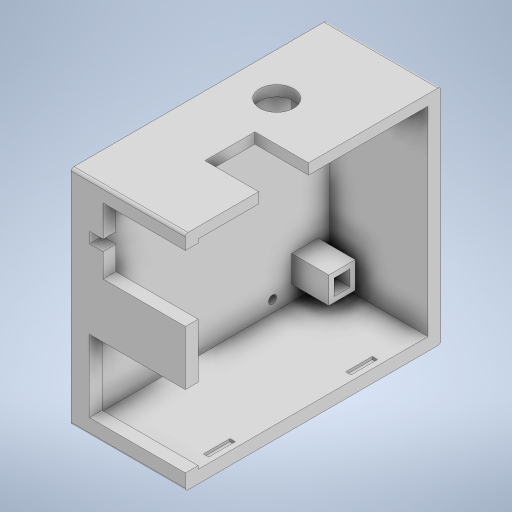
# Autodesk Inventor part: Enclosure_Top_v2
Saved by Autodesk Inventor 2023 (Build 270158030, 158C)
## iProperties
Created: 2023-12-07
Part Number: Enclosure_Top_v2
Material: Generic
Document SubType Name: Sheet Metal
Designer: Fabian
Density: 1 g/cm^3
Sheet Metal Rule: Default_mm
Appearance: Default
Author: Fabian
Autodesk Inventor part; units mm, degrees
ref_plane "YZ Plane" through (0, 0, 0) normal (1, 0, 0) x (0, 1, 0)
ref_plane "XZ Plane" through (0, 0, 0) normal (0, 1, 0) x (-1, 0, 0)
ref_plane "XY Plane" through (0, 0, 0) normal (0, 0, 1) x (1, 0, 0)
sketch "Sketch1" plane through (0, 0, 0) normal (1, 0, 0) x (0, 1, 0)
  line L0 (10.2141, 17.9541) -> (-31.7859, 17.9541)
  line L1 (-31.7859, 17.9541) -> (-31.7859, -30.1559)
  line L2 (-31.7859, -30.1559) -> (10.2141, -30.1559)
  line L3 (10.2141, -30.1559) -> (10.2141, 17.9541)
  point P0 (0, 0)
  dimension "d0" = 42
  dimension "d1" = 48.11
  constraints: 8 end point, 2 parallel, 1 horizontal, 1 perpendicular
  measures "d0" distance of L2.end L1.end
  measures "d1" distance of L1.end L0.end
extrude "BasePlate" add sketch "Sketch1" along normal blind 3
sketch "Sketch2" plane through (3, 0, 0) normal (1, 0, 0) x (0, 0, -1)
  point P0 (0, 0)
sketch "Sketch3" plane through (3, 0, 0) normal (1, 0, 0) x (0, 0, -1)
  line L0 (30.1559, 10.2141) -> (-17.9541, 10.2141) projected
  line L1 (-17.9541, -31.7859) -> (30.1559, -31.7859) projected
  line L2 (-17.9541, 10.2141) -> (30.1559, 10.2141)
  line L3 (30.1559, 10.2141) -> (30.1559, -31.7859)
  line L4 (30.1559, -31.7859) -> (-17.9541, -31.7859)
  line L5 (-17.9541, -31.7859) -> (-17.9541, 10.2141)
  line L6 (-15.5541, 8.2141) -> (27.7559, 8.2141)
  line L7 (27.7559, 8.2141) -> (27.7559, -29.3859)
  line L8 (27.7559, -29.3859) -> (-15.5541, -29.3859)
  line L9 (-15.5541, -29.3859) -> (-15.5541, 8.2141)
  point P0 (0, 0)
  point P1 (-17.9541, -10.7859)
  dimension "d4" = 2
  dimension "d5" = 2.4
  dimension "d6" = 2.4
  dimension "d7" = 2.4
  constraints: 16 end point, 4 parallel, 2 horizontal, 2 perpendicular, 1 midpoint
  measures "d4" distance between parallel lines of L0 L6
  measures "d5" distance between parallel lines of L1 L8
  measures "d6" distance from line of point (-17.954, -10.786) L9
  measures "d7" distance between parallel lines of L3 L7
extrude "Walls" add sketch "Sketch3" along normal blind 18.5
sketch "Sketch4" plane through (21.5, 0, 0) normal (1, 0, 0) x (0, 0, -1)
  line L0 (30.1559, 10.2141) -> (-17.9541, 10.2141) projected
  line L1 (-15.5541, 8.2141) -> (27.7559, 8.2141) projected
  line L2 (-4.1541, 10.2141) -> (5.2459, 10.2141)
  line L3 (5.2459, 10.2141) -> (5.2459, 8.2141)
  line L4 (5.2459, 8.2141) -> (-4.1541, 8.2141)
  line L5 (-4.1541, 8.2141) -> (-4.1541, 10.2141)
  line L6 (-17.9541, 10.2141) -> (-17.9541, -31.7859) projected
  point P0 (0, 0)
  point P1 (-4.1541, 9.2141)
  point P2 (5.2459, 10.2141)
  dimension "d10" = 9.4
  dimension "d11" = 13.8
  constraints: 8 end point, 2 parallel, 2 point on line, 1 horizontal, 1 midpoint, 1 perpendicular
  measures "d10" distance of L3.end L4.end
  measures "d11" distance from line of point (-4.154, 9.214) L6
extrude "USB-C" cut sketch "Sketch4" against normal blind 10.1
sketch "Sketch5" plane through (21.5, 0, 0) normal (1, 0, 0) x (0, 0, -1)
  line L0 (-17.9541, 10.2141) -> (-17.9541, -31.7859) projected
  line L1 (-15.5541, -29.3859) -> (-15.5541, 8.2141) projected
  line L2 (-17.9541, -4.8859) -> (-15.5541, -4.8859)
  line L3 (-15.5541, -4.8859) -> (-15.5541, 7.5141)
  line L4 (-15.5541, 7.5141) -> (-17.9541, 7.5141)
  line L5 (-17.9541, 7.5141) -> (-17.9541, -4.8859)
  line L6 (-4.1541, 10.2141) -> (-17.9541, 10.2141) projected
  point P0 (0, 0)
  point P1 (-16.7541, 7.5141)
  point P2 (-17.9541, 7.5141)
  point P3 (-15.5541, -4.8859)
  dimension "d14" = 12.4
  dimension "d15" = 2.7
  constraints: 8 end point, 2 parallel, 2 point on line, 1 horizontal, 1 midpoint, 1 perpendicular
  measures "d14" distance of L3.end L2.end
  measures "d15" distance from line of L6 point (-16.754, 7.514)
extrude "PowerConnector1" cut sketch "Sketch5" against normal blind 15.5
sketch "Sketch6" plane through (6, 0, 0) normal (1, 0, 0) x (0, 0, -1)
  line L0 (-17.9541, 10.2141) -> (-17.9541, -31.7859) projected
  line L1 (-17.9541, -0.3859) -> (-15.5541, -0.3859)
  line L2 (-15.5541, -0.3859) -> (-15.5541, 1.6141)
  line L3 (-15.5541, 1.6141) -> (-17.9541, 1.6141)
  line L4 (-17.9541, 1.6141) -> (-17.9541, -0.3859)
  line L5 (-17.9541, 7.5141) -> (-15.5541, 7.5141) projected
  point P0 (0, 0)
  dimension "d18" = 2.4
  dimension "d19" = 2
  dimension "d20" = 5.9
  constraints: 8 end point, 2 parallel, 1 horizontal, 1 perpendicular, 1 point on line
  measures "d18" distance of L3.end L2.end
  measures "d19" distance of L1.end L2.end
  measures "d20" distance between parallel lines of L5 L3
extrude "PowerConnector2" cut sketch "Sketch6" against normal blind 2.5
sketch "Sketch8" plane through (21.5, 0, 0) normal (1, 0, 0) x (0, 0, -1)
  line L0 (-17.9541, 10.2141) -> (-17.9541, -31.7859) projected
  line L1 (-15.5541, 8.2141) -> (-15.5541, -29.3859) projected
  line L2 (-17.9541, -28.7859) -> (-15.5541, -28.7859)
  line L3 (-15.5541, -28.7859) -> (-15.5541, -15.1859)
  line L4 (-15.5541, -15.1859) -> (-17.9541, -15.1859)
  line L5 (-17.9541, -15.1859) -> (-17.9541, -28.7859)
  line L6 (-17.9541, -31.7859) -> (30.1559, -31.7859) projected
  point P0 (0, 0)
  dimension "d23" = 13.6
  dimension "d24" = 3
  constraints: 8 end point, 2 parallel, 2 point on line, 1 horizontal, 1 perpendicular
  measures "d23" distance of L3.end L2.end
  measures "d24" distance between parallel lines of L6 L2
extrude "RJ-12" cut sketch "Sketch8" against normal blind 18.1
fillet "Fillet1" radius 0.5 4 edges at (10.75, 10.2141, 17.9541) (10.75, -31.7859, 17.9541) (10.75, 10.2141, -30.1559) (10.75, -31.7859, -30.1559)
sketch "Sketch9" plane through (0, 0, 0) normal (-1, 0, 0) x (0, 0, 1)
  line L0 (-24.5559, -25.4859) -> (-21.5559, -25.4859)
  line L1 (-21.5559, -25.4859) -> (-21.5559, -22.4859)
  line L2 (-21.5559, -22.4859) -> (-24.5559, -22.4859)
  line L3 (-24.5559, -22.4859) -> (-24.5559, -25.4859)
  line L4 (-30.1559, -31.2859) -> (-30.1559, 9.7141) projected
  line L5 (17.4541, -31.7859) -> (-29.6559, -31.7859) projected
  point P0 (0, 0)
  point P1 (-24.5559, -23.9859)
  dimension "d28" = 3
  dimension "d29" = 3
  dimension "d30" = 5.6
  dimension "d31" = 6.3
  constraints: 8 end point, 2 parallel, 1 horizontal, 1 midpoint, 1 perpendicular
  measures "d28" distance of L2.end L1.end
  measures "d29" distance of L1.end L0.end
  measures "d30" distance from line of L4 point (-24.556, -23.986)
  measures "d31" distance between parallel lines of L5 L0
extrude "ZBButton" cut sketch "Sketch9" against normal blind 3
sketch "Sketch10" plane through (0, 0, 0) normal (-1, 0, 0) x (0, 0, 1)
  line L0 (-24.5559, 0.9141) -> (-21.5559, 0.9141)
  line L1 (-21.5559, 0.9141) -> (-21.5559, 3.9141)
  line L2 (-21.5559, 3.9141) -> (-24.5559, 3.9141)
  line L3 (-24.5559, 3.9141) -> (-24.5559, 0.9141)
  line L4 (-30.1559, -31.2859) -> (-30.1559, 9.7141) projected
  line L5 (-29.6559, 10.2141) -> (17.4541, 10.2141) projected
  point P0 (0, 0)
  point P1 (-24.5559, 2.4141)
  dimension "d34" = 3
  dimension "d35" = 3
  dimension "d36" = 5.6
  dimension "d37" = 6.3
  constraints: 8 end point, 2 parallel, 1 horizontal, 1 midpoint, 1 perpendicular
  measures "d34" distance of L2.end L1.end
  measures "d35" distance of L1.end L0.end
  measures "d36" distance from line of L4 point (-24.556, 2.414)
  measures "d37" distance between parallel lines of L5 L2
extrude "ResetButton" cut sketch "Sketch10" against normal blind 3
sketch "Sketch11" plane through (3, 0, 0) normal (1, 0, 0) x (0, 0, -1)
  line L0 (25.5559, 4.9141) -> (20.5559, 4.9141)
  line L1 (20.5559, 4.9141) -> (20.5559, -0.0859)
  line L2 (20.5559, -0.0859) -> (25.5559, -0.0859)
  line L3 (25.5559, -0.0859) -> (25.5559, 4.9141)
  line L4 (21.5559, 3.9141) -> (24.5559, 3.9141) projected
  line L5 (24.5559, 3.9141) -> (24.5559, 0.9141) projected
  line L6 (25.5559, -21.4859) -> (20.5559, -21.4859)
  line L7 (20.5559, -21.4859) -> (20.5559, -26.4859)
  line L8 (20.5559, -26.4859) -> (25.5559, -26.4859)
  line L9 (25.5559, -26.4859) -> (25.5559, -21.4859)
  line L10 (24.5559, -22.4859) -> (24.5559, -25.4859) projected
  line L11 (21.5559, -22.4859) -> (24.5559, -22.4859) projected
  line L12 (24.5559, 0.9141) -> (21.5559, 0.9141) projected
  line L13 (24.5559, 3.9141) -> (21.5559, 3.9141)
  line L14 (21.5559, 3.9141) -> (21.5559, 0.9141)
  line L15 (21.5559, 0.9141) -> (24.5559, 0.9141)
  line L16 (24.5559, 0.9141) -> (24.5559, 3.9141)
  line L17 (21.5559, -25.4859) -> (21.5559, -22.4859) projected
  line L18 (24.5559, -22.4859) -> (21.5559, -22.4859)
  line L19 (21.5559, -22.4859) -> (21.5559, -25.4859)
  line L20 (21.5559, -25.4859) -> (24.5559, -25.4859)
  line L21 (24.5559, -25.4859) -> (24.5559, -22.4859)
  point P0 (0, 0)
  point P1 (23.0559, -22.4859)
  dimension "d40" = 5
  dimension "d41" = 5
  dimension "d42" = 1
  dimension "d43" = 1
  dimension "d44" = 5
  dimension "d45" = 5
  dimension "d46" = 1
  dimension "d47" = 1
  constraints: 32 end point, 8 parallel, 4 horizontal, 4 perpendicular, 1 midpoint
  measures "d40" distance of L2.end L1.end
  measures "d41" distance of L1.end L0.end
  measures "d42" distance between parallel lines of L4 L0
  measures "d43" distance between parallel lines of L3 L5
  measures "d44" distance of L8.end L7.end
  measures "d45" distance of L7.end L6.end
  measures "d46" distance between parallel lines of L9 L10
  measures "d47" distance from line of point (23.056, -22.486) L6
extrude "ButtonFuehrung" add sketch "Sketch11" along normal blind 7
sketch "Sketch12" plane through (0, 0, 0) normal (-1, 0, 0) x (0, 0, 1)
  circle A0 centre (-16.9559, -27.1859) radius 0.75
  line L0 (17.4541, -31.7859) -> (-29.6559, -31.7859) projected
  line L1 (-30.1559, -31.2859) -> (-30.1559, 9.7141) projected
  point P0 (0, 0)
  dimension "d50" = 1.5
  dimension "d51" = 4.6
  dimension "d52" = 13.2
  constraints: 1 centre point
  measures "d50" diameter of A0
  measures "d51" distance from line of L0 A0.centre
  measures "d52" distance from line of L1 A0.centre
extrude "LED" cut sketch "Sketch12" against normal blind 3
sketch "Sketch13" plane through (11.4, 10.2141, 4.1541) normal (0, 1, 0) x (1, 0, 0)
  circle A0 centre (-3.4, 16.91) radius 3.2
  line L0 (-11.4, 33.81) -> (-11.4, -13.3) projected
  line L1 (10.1, 34.31) -> (-11.4, 34.31) projected
  point P0 (-11.4, 4.1541)
  dimension "d55" = 6.4
  dimension "d56" = 8
  dimension "d57" = 17.4
  constraints: 1 centre point
  measures "d55" diameter of A0
  measures "d56" distance from line of L0 A0.centre
  measures "d57" distance from line of L1 A0.centre
extrude "Antenna" cut sketch "Sketch13" against normal blind 2
sketch "Sketch14" plane through (3, 8.2141, -27.7559) normal (0, -1, 0) x (1, 0, 0)
  line L0 (17.5, 40.31) -> (16.5, 40.31)
  line L1 (16.5, 40.31) -> (16.5, 35.31)
  line L2 (16.5, 35.31) -> (17.5, 35.31)
  line L3 (17.5, 35.31) -> (17.5, 40.31)
  line L4 (18.5, 43.31) -> (18.5, 31.91) projected
  point P0 (-3, 27.7559)
  point P1 (17.5, 37.81)
  dimension "d60" = 1
  dimension "d61" = 5
  dimension "d62" = 1
  dimension "d63" = 5.5
  constraints: 8 end point, 2 parallel, 1 horizontal, 1 midpoint, 1 perpendicular
  measures "d60" distance of L2.end L1.end
  measures "d61" distance of L1.end L0.end
  measures "d62" distance between parallel lines of L4 L3
  measures "d63" vertical distance of L4.start point (17.5, 37.81)
extrude "Extrusion12" cut sketch "Sketch14" against normal blind 0.5
sketch "Sketch15" plane through (3, 8.2141, -27.7559) normal (0, -1, 0) x (1, 0, 0)
  line L0 (17.5, 13.5) -> (16.5, 13.5)
  line L1 (16.5, 13.5) -> (16.5, 8.5)
  line L2 (16.5, 8.5) -> (17.5, 8.5)
  line L3 (17.5, 8.5) -> (17.5, 13.5)
  line L4 (18.5, 22.51) -> (18.5, 0) projected
  line L5 (0, 0) -> (18.5, 0) projected
  point P0 (-3, 27.7559)
  point P1 (17.5, 11)
  dimension "d66" = 1
  dimension "d67" = 5
  dimension "d68" = 1
  dimension "d69" = 11
  constraints: 8 end point, 2 parallel, 1 horizontal, 1 midpoint, 1 perpendicular
  measures "d66" distance of L2.end L1.end
  measures "d67" distance of L1.end L0.end
  measures "d68" distance from line of L4 point (17.5, 11)
  measures "d69" distance from line of L5 point (17.5, 11)
extrude "Extrusion13" cut sketch "Sketch15" against normal blind 0.5
sketch "Sketch16" plane through (3, -29.3859, 15.5541) normal (0, 1, 0) x (1, 0, 0)
  line L0 (17.5, 8) -> (16.5, 8)
  line L1 (16.5, 8) -> (16.5, 3)
  line L2 (16.5, 3) -> (17.5, 3)
  line L3 (17.5, 3) -> (17.5, 8)
  line L4 (18.5, 43.31) -> (18.5, 0) projected
  line L5 (0, 0) -> (18.5, 0) projected
  point P0 (-3, 15.5541)
  point P1 (17.5, 5.5)
  dimension "d72" = 1
  dimension "d73" = 5
  dimension "d74" = 1
  dimension "d75" = 5.5
  constraints: 8 end point, 2 parallel, 1 horizontal, 1 midpoint, 1 perpendicular
  measures "d72" distance of L2.end L1.end
  measures "d73" distance of L1.end L0.end
  measures "d74" distance between parallel lines of L4 L3
  measures "d75" distance from line of L5 point (17.5, 5.5)
extrude "Extrusion14" cut sketch "Sketch16" against normal blind 0.5
sketch "Sketch17" plane through (3, -29.3859, 15.5541) normal (0, 1, 0) x (1, 0, 0)
  line L0 (17.5, 34.81) -> (16.5, 34.81)
  line L1 (16.5, 34.81) -> (16.5, 29.81)
  line L2 (16.5, 29.81) -> (17.5, 29.81)
  line L3 (17.5, 29.81) -> (17.5, 34.81)
  line L4 (18.5, 43.31) -> (18.5, 0) projected
  line L5 (0, 43.31) -> (18.5, 43.31) projected
  point P0 (-3, 15.5541)
  point P1 (17.5, 32.31)
  dimension "d78" = 1
  dimension "d79" = 5
  dimension "d80" = 1
  dimension "d81" = 11
  constraints: 8 end point, 2 parallel, 1 horizontal, 1 midpoint, 1 perpendicular
  measures "d78" distance of L2.end L1.end
  measures "d79" distance of L1.end L0.end
  measures "d80" distance between parallel lines of L4 L3
  measures "d81" distance from line of L5 point (17.5, 32.31)
extrude "Extrusion15" cut sketch "Sketch17" against normal blind 0.5
equation "\"BendRadius\" = Thickness"
equation "\"BendReliefWidth\" = Thickness"
equation "\"BendReliefDepth\" = 0.5 * Thickness"
equation "\"CornerReliefSize\" = 4 * Thickness"
equation "\"MinimumRemnant\" = 2 * Thickness"
equation "\"TransitionRadius\" = BendRadius"
equation "\"JacobiRadiusSize\" = BendRadius"
equation "\"GapSize\" = Thickness"
equation "\"Thickness\" = 0.5"
body "Solid1"
